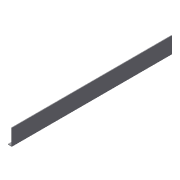
# Autodesk Inventor part: ISPFrame
Saved by Autodesk Inventor 2015 (Build 190159000, 159)
## iProperties
Created: 2015-03-06
Part Number: ISPFrame
Material: Generic
Document SubType Name: Modeling
Designer: Kyle
Density: 1 g/cm^3
Appearance: Default
Author: Kyle
Autodesk Inventor part; units mm, degrees
ref_plane "YZ Plane" through (0, 0, 0) normal (1, 0, 0) x (0, 1, 0)
ref_plane "XZ Plane" through (0, 0, 0) normal (0, 1, 0) x (-1, 0, 0)
ref_plane "XY Plane" through (0, 0, 0) normal (0, 0, 1) x (1, 0, 0)
sketch "Sketch1" plane through (0, 0, 0) normal (0, 0, 1) x (1, 0, 0)
  line L0 (0, 0) -> (19.05, 0)
  line L1 (0, 0) -> (19.05, 0) construction
  line L2 (19.05, 0) -> (19.05, 82.55)
  line L3 (19.05, 82.55) -> (15.875, 82.55)
  line L4 (15.875, 82.55) -> (15.875, 3.175)
  line L5 (15.875, 3.175) -> (0, 3.175)
  line L6 (0, 3.175) -> (0, 0)
  dimension "d0" = 19.05
  dimension "d1" = 0
  dimension "d2" = 82.55
  dimension "d3" = 90
  dimension "d4" = 3.175
  dimension "d5" = 79.375
  constraints: 14 end point, 4 perpendicular, 2 horizontal, 1 collinear, 1 vertical
  measures "d0" distance of L0.start L0.end
  measures "d1" distance between parallel lines of L0 L1
  measures "d2" distance of L0.end L2.end
  measures "d3" angle of L2 L0
  measures "d4" distance of L2.end L3.end
  measures "d5" distance of L3.end L4.end
sketch "Sketch2" plane through (0, 0, 0) normal (0, 0, 1) x (1, 0, 0)
  point P0 (0, 0)
extrude "Extrusion3" add sketch "Sketch1" along normal blind 809.625
body "Solid3"
